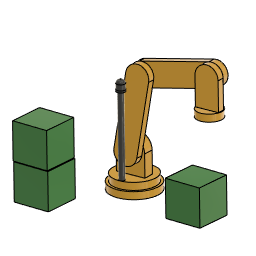
Robot (Autodesk Fusion 360 design; units mm, degrees)
Autodesk Fusion 360 part; units mm, degrees
sketch "Sketch1" plane through (0, 0, 0) normal (0, 0, 1) x (1, 0, 0) in component "Box"
  line L0 (50, 50) -> (-50, 50)
  line L1 (-50, 50) -> (-50, -50)
  line L2 (-50, -50) -> (50, -50)
  line L3 (50, -50) -> (50, 50)
  line L4 (50, 50) -> (-50, -50) construction
  line L5 (-50, 50) -> (50, -50) construction
  dimension "d1" = 100
  dimension "d2" = 100
  constraint horizontal L0
  constraint perpendicular L0 L1
  constraint parallel L0 L2
  constraint parallel L1 L3
  constraint coincident L4 origin
  constraint coincident L5 origin
  measures "d1" distance of L1.end L2.end
  measures "d2" distance of L0.end L1.end
extrude "Extrude1" add sketch "Sketch1" along normal blind 100 makes body 1 in component "Box"
sketch "Sketch1 (2)" plane through (0, 0, 0) normal (0, 0, 1) x (1, 0, 0) in component "Base"
  circle A0 centre (139.9127, 198.8015) radius 60
  dimension "d5" = 120
  measures "d5" diameter of A0
extrude "Extrude1'" add sketch "Sketch1 (2)" along normal blind 40 separate body makes body 2 in component "Base"
sketch "Sketch2" plane through (0, 0, 40) normal (0, 0, 1) x (-1, 0, 0) in component "Base"
  circle A0 centre (-139.9127, -198.8015) radius 60
  line L0 (-124.9127, -238.8015) -> (-154.9127, -238.8015)
  line L1 (-154.9127, -238.8015) -> (-154.9127, -158.8015)
  line L2 (-154.9127, -158.8015) -> (-124.9127, -158.8015)
  line L3 (-124.9127, -158.8015) -> (-124.9127, -238.8015)
  line L4 (-124.9127, -238.8015) -> (-154.9127, -158.8015) construction
  line L5 (-154.9127, -238.8015) -> (-124.9127, -158.8015) construction
  point P0 (-139.9127, -198.8015)
  dimension "d8" = 30
  dimension "d9" = 80
  constraint horizontal L0
  constraint perpendicular L0 L1
  constraint parallel L0 L2
  constraint parallel L1 L3
  constraint coincident L4 P0
  constraint coincident L5 P0
  constraint coincident P0 A0.centre
  measures "d8" distance of L1.end L2.end
  measures "d9" distance of L0.end L1.end
extrude "Extrude2" add sketch "Sketch2" along normal blind 100 contours L0 L1 L2 L3 bodies 2 in component "Base"
fillet "Fillet1" radius 40 2 edges at (139.9127, 238.8015, 140) (139.9127, 158.8015, 140) on bodies 2 in component "Base"
sketch "Sketch1 (3)" plane through (154.9127, 0, 0) normal (1, 0, 0) x (0, 1, 0) in component "Liink"
  arc A0 (238.8015, 100) -> (158.8015, 100) centre (198.8015, 100) ccw
  line L0 (158.8015, 100) -> (158.8015, 40)
  line L1 (158.8015, 40) -> (238.8015, 40)
  line L2 (238.8015, 40) -> (238.8015, 100)
  circle A1 centre (198.8015, 100) radius 32.5
  circle A2 centre (198.8015, 300) radius 32.5
  line L3 (166.3015, 300) -> (166.3015, 100)
  line L4 (231.3015, 300) -> (231.3015, 100)
  dimension "d14" = 65
  dimension "d15" = 65
  dimension "d16" = 200
  constraint concentric A0 A1
  constraint vertical A0.centre A2.centre
  constraint coincident A2 L3.start
  constraint tangent A2 L3
  constraint coincident A1 L3.end
  constraint tangent A1 L3
  constraint coincident A2 L4.start
  constraint tangent A2 L4
  constraint coincident A1 L4.end
  constraint tangent A1 L4
  measures "d14" diameter of A1
  measures "d15" diameter of A2
  measures "d16" distance of A0.centre A2.centre
extrude "Extrude1''" add sketch "Sketch1 (3)" along normal blind 20 separate body contours A0 A1 L3 L4 | A0 A2 L3 L4 | A2 | A1 makes body 3 in component "Liink"
move_face "OffsetFaces1" offset -20 1 faces at (121.2282, 198.9998, 0) on bodies 2 in component "Base"
sketch "Sketch1 (4)" plane through (0, 0, 20) normal (0, 0, -1) x (1, 0, 0) in component "Ground"
  circle A0 centre (139.9127, -198.8015) radius 60
  circle A1 centre (139.9127, -198.8015) radius 67.5
  dimension "d20" = 135
  constraint concentric A0 A1
  measures "d20" diameter of A1
extrude "Extrude1'''" add sketch "Sketch1 (4)" along normal blind 20 separate body contours A0 | A1 makes body 4 in component "Ground"
sketch "Sketch1 (5)" plane through (154.9127, 0, 0) normal (1, 0, 0) x (0, 1, 0) in component "Grab"
  line L0 (166.3015, 450) -> (166.3015, 250)
  arc A0 (166.3015, 250) -> (231.3015, 250) centre (198.8015, 250) ccw
  line L1 (231.3015, 250) -> (231.3015, 450)
  arc A1 (231.3015, 450) -> (166.3015, 450) centre (198.8015, 450) ccw
  circle A2 centre (198.8015, 450) radius 32.5
  line L2 (198.8015, 482.5) -> (119.7676, 482.5)
  line L3 (119.7676, 482.5) -> (119.7676, 417.5)
  line L4 (119.7676, 417.5) -> (198.8015, 417.5)
  line L5 (198.8015, 417.5) -> (198.8015, 482.5)
  constraint concentric A1 A2
  constraint coincident L1.end A2
  constraint horizontal L2
  constraint vertical L3
  constraint horizontal L4
  constraint vertical L5
  constraint midpoint A1 L2.start
  constraint coincident A2 L4.end
extrude "Extrude1''''" add sketch "Sketch1 (5)" along normal blind 20 separate body contours L0 A2 L4 | L0 A1 A2 L2 L3 L4 | A1 A2 L5 | A1 A2 L5 makes body 5 in component "Grab"
sketch "Sketch2 (2)" plane through (0, 119.7676, 0) normal (0, -1, 0) x (1, 0, 0) in component "Grab"
  line L0 (154.9127, 482.5) -> (154.9127, 417.5)
  line L1 (154.9127, 417.5) -> (174.9127, 417.5)
  line L2 (174.9127, 417.5) -> (174.9127, 482.5)
  line L3 (174.9127, 482.5) -> (154.9127, 482.5)
  line L4 (154.9127, 482.5) -> (174.9127, 417.5) construction
  circle A0 centre (164.9127, 450) radius 35
  dimension "d25" = 70
  constraint coincident L0.start L3.end
  constraint coincident L1.end L2.start
  constraint midpoint L4 A0.centre
  measures "d25" diameter of A0
extrude "Extrude2'" add sketch "Sketch2 (2)" along normal blind 20 contours L0 L1 L2 L3 | A0 bodies 5 in component "Grab"
move_face "MoveFace1" by (24.2333, 26.6566, 0) 1 faces at (-16.6667, 16.6667, 0) on bodies 1 in component "Box"
sketch "Sketch1 (6)" plane through (0, 0, 0) normal (0, 0, -1) x (1, 0, 0) in component "helper"
  circle A0 centre (139.9127, -198.8015) radius 67.5
  circle A1 centre (139.9127, -198.8015) radius 290.62
  constraint concentric A0 A1
extrude "Extrude1'''''" add sketch "Sketch1 (6)" against normal blind 175 separate body contours A0 | A1 makes body 6 in component "helper"
sketch "Sketch1 (7)" plane through (0, 0, 40) normal (0, 0, 1) x (-1, 0, 0) in component "pole"
  line L0 (-124.9127, -158.8015) -> (-124.9127, -238.8015)
  line L1 (-124.9127, -238.8015) -> (-154.9127, -238.8015)
  line L2 (-154.9127, -238.8015) -> (-154.9127, -158.8015)
  line L3 (-154.9127, -158.8015) -> (-124.9127, -158.8015)
  circle A0 centre (-139.9127, -198.8015) radius 60
  circle A1 centre (-191.2717, -199.7385) radius 8.2017
extrude "Extrude1''''''" add sketch "Sketch1 (7)" along normal blind 220 separate body contours A1 makes body 7 in component "pole"
sketch "Sketch2 (3)" plane through (0, 0, 260) normal (0, 0, 1) x (-1, 0, 0) in component "pole"
  circle A0 centre (-191.2717, -199.7385) radius 8.2017
  circle A1 centre (-191.2717, -199.7385) radius 11.9048
  constraint concentric A0 A1
extrude "Extrude2''" add sketch "Sketch2 (3)" along normal blind 5 contours A0 | A1 bodies 7 in component "pole"
sketch "Sketch1 (8)" plane through (0, 0, 265) normal (0, 0, 1) x (-1, 0, 0) in component "LIGHT"
  circle A0 centre (-191.2717, -199.7385) radius 11.9048
  circle A1 centre (-191.2717, -199.7385) radius 11.9048
  constraint concentric A0 A1
extrude "Extrude1'''''''" add sketch "Sketch1 (8)" along normal blind 25 separate body makes body 8 in component "LIGHT"
fillet "Fillet1'" radius 10 1 edges at (202.3709, 204.0435, 290) on bodies 8 in component "LIGHT"
component "Box" placed x (1, 0, 0) y (0, 1, 0) z (0, 0, 1) at (18.5789, 19.3867, 0)
component "Box" placed x (1, 0, 0) y (0, 1, 0) z (0, 0, 1) at (360, 150, 0)
component "Box" placed x (1, 0, 0) y (0, 1, 0) z (0, 0, 1) at (14.6534, 22.1014, 100)
component "Base" placed x (0.058506, -0.998287, 0) y (0.998287, 0.058506, 0) z (0, 0, 1) at (-66.734, 326.8435, 0)
component "Liink" placed x (0.058506, -0.998287, 0) y (0.994958, 0.058311, -0.081593) z (0.081454, 0.004774, 0.996666) at (-74.2177, 326.4049, 16.5543)
component "Ground" placed x (1, 0, 0) y (0, 1, 0) z (0, 0, 1) at (0, 0, 0)
component "Liink" placed x (0.058506, -0.998287, 0) y (0.306999, 0.017992, -0.95154) z (0.94991, 0.055671, 0.307526) at (-9.1753, 350.2511, 457.7481)
component "Grab" placed x (0.058506, -0.998287, 0) y (0, 0, 1) z (-0.998287, -0.058506, 0) at (787.2288, 376.8913, 162.0368)
component "helper" placed x (1, 0, 0) y (0, 1, 0) z (0, 0, 1) at (0, 0, 86.8043)
component "pole" placed x (1, 0, 0) y (0, 1, 0) z (0, 0, 1) at (0, 0, 0) in component "Base"
component "LIGHT" placed x (1, 0, 0) y (0, 1, 0) z (0, 0, 1) at (0, 0, 0) in component "Base"
